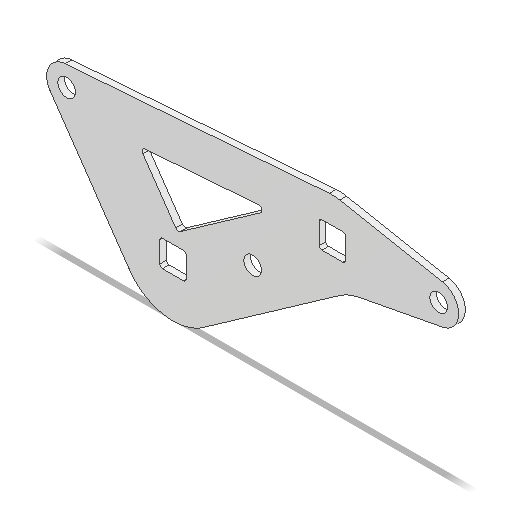
# Autodesk Inventor part: Gearbox
Saved by Autodesk Inventor 2025.2 (Build 292293000, 293)
## iProperties
Created: 2025-02-16
Part Number: Gearbox
Material: Acetal Resin, White
Document SubType Name: Modeling
Designer: avere
Density: 1.425 g/cm^3
Appearance: Smooth - White
Author: avere
Autodesk Inventor part; units mm, degrees
ref_plane "YZ Plane" through (0, 0, 0) normal (1, 0, 0) x (0, 1, 0)
ref_plane "XZ Plane" through (0, 0, 0) normal (0, 1, 0) x (-1, 0, 0)
ref_plane "XY Plane" through (0, 0, 0) normal (0, 0, 1) x (1, 0, 0)
sketch "Sketch1" plane through (0, 0, 0) normal (0, 0, 1) x (1, 0, 0)
  line L0 (35.5854, -19.7457) -> (40.6146, -19.7457)
  line L1 (41.2496, -20.3807) -> (41.2496, -25.4099)
  line L2 (40.6146, -26.0449) -> (35.5854, -26.0449)
  line L3 (34.9504, -25.4099) -> (34.9504, -20.3807)
  line L4 (34.9504, -19.7457) -> (41.2496, -26.0449) construction
  line L5 (41.2496, -19.7457) -> (34.9504, -26.0449) construction
  line L6 (73.6854, 3.1496) -> (78.7146, 3.1496)
  line L7 (79.3496, 2.5146) -> (79.3496, -2.5146)
  line L8 (78.7146, -3.1496) -> (73.6854, -3.1496)
  line L9 (73.0504, -2.5146) -> (73.0504, 2.5146)
  line L10 (73.0504, 3.1496) -> (79.3496, -3.1496) construction
  line L11 (79.3496, 3.1496) -> (73.0504, -3.1496) construction
  arc A0 (35.5854, -19.7457) -> (34.9504, -20.3807) centre (35.5854, -20.3807) ccw
  arc A1 (34.9504, -25.4099) -> (35.5854, -26.0449) centre (35.5854, -25.4099) ccw
  arc A2 (40.6146, -26.0449) -> (41.2496, -25.4099) centre (40.6146, -25.4099) ccw
  arc A3 (41.2496, -20.3807) -> (40.6146, -19.7457) centre (40.6146, -20.3807) ccw
  arc A4 (73.0504, -2.5146) -> (73.6854, -3.1496) centre (73.6854, -2.5146) ccw
  arc A5 (73.6854, 3.1496) -> (73.0504, 2.5146) centre (73.6854, 2.5146) ccw
  arc A6 (79.3496, 2.5146) -> (78.7146, 3.1496) centre (78.7146, 2.5146) ccw
  arc A7 (78.7146, -3.1496) -> (79.3496, -2.5146) centre (78.7146, -2.5146) ccw
  arc A8 (12.3428, 4.7491) -> (8.7773, -2.7007) centre (12.7, 0) ccw
  arc A9 (77.9859, 9.3561) -> (75.4856, 9.4982) centre (76.2, 0) ccw
  arc A10 (27.6395, -30.0972) -> (45.4023, -33.2859) centre (38.1, -22.8953) ccw
  line L12 (12.3428, 4.7491) -> (75.4856, 9.4982)
  line L13 (8.7773, -2.7007) -> (27.6395, -30.0972)
  line L14 (45.4023, -33.2859) -> (77.7633, -10.5433)
  circle A11 centre (12.7, 0) radius 2.0955
  circle A12 centre (101.6, 0) radius 2.0955
  arc A13 (102.493, -4.678) -> (102.493, 4.678) centre (101.6, 0) ccw
  line L15 (77.9859, 9.3561) -> (102.493, 4.678)
  line L16 (102.493, -4.678) -> (82.6844, -8.4592)
  arc A14 (82.6844, -8.4592) -> (77.7633, -10.5433) centre (85.0656, -20.934) ccw
  line L17 (31.4974, -3.3622) -> (58.4855, -1.3323)
  line L18 (39.8718, -16.2172) -> (59.0014, -2.7733)
  line L19 (30.9032, -4.6038) -> (38.7616, -16.0179)
  arc A15 (31.4974, -3.3622) -> (30.9032, -4.6038) centre (31.5569, -4.1537) ccw
  arc A16 (38.7616, -16.0179) -> (39.8718, -16.2172) centre (39.4154, -15.5677) ccw
  arc A17 (59.0014, -2.7733) -> (58.4855, -1.3323) centre (58.545, -2.1239) ccw
  circle A18 centre (57.15, -14.5521) radius 2.0955
  point P0 (76.2, 0)
  point P1 (79.9995, -8.9717)
  point P2 (38.1, -22.8953)
  dimension "d7" = 6.2992
  dimension "d8" = 6.2992
  dimension "d12" = 6.2992
  dimension "d13" = 6.2992
  dimension "d16" = 19.05
  dimension "d17" = 25.4
  dimension "d21" = 4.191
  dimension "d22" = 63.5
  dimension "d23" = 4.7625
  dimension "d24" = 4.191
  dimension "d25" = 9.525
  dimension "d26" = 25.4
  dimension "d27" = 12.7
  dimension "d28" = 9.525
  dimension "d31" = 17.145
  dimension "d32" = 17.145
  dimension "d33" = 0.7937
  dimension "d34" = 4.191
  dimension "d38" = 8.5725
  constraints: 40 end point, 34 tangent, 32 point on circle, 19 centre point, 18 point on line, 9 equal radius, 7 parallel, 4 midpoint, 3 coincident, 2 horizontal, 2 horizontal alignment, 2 perpendicular, 2 other
  measures "d7" distance of L10.end L11.end
  measures "d8" distance of L11.start L10.end
  measures "d12" distance of L5.end L4.start
  measures "d13" distance of L4.end L5.end
  measures "d16" diameter of A9
  measures "d17" diameter of A10
  measures "d21" diameter of A11
  measures "d22" distance of A9.centre A8.centre
  measures "d23" radius of A8
  measures "d24" diameter of A12
  measures "d25" diameter of A13
  measures "d26" distance of A12.centre A9.centre
  measures "d27" radius of A14
  measures "d28" distance between parallel lines of L17 L12
  measures "d31" distance between parallel lines of L14 L18
  measures "d32" distance between parallel lines of L13 L19
  measures "d33" radius of A15
  measures "d34" diameter of A18
  measures "d38" distance from line of L18 A18.centre
extrude "Extrusion1" add sketch "Sketch1" along normal blind 1.5875
body "Solid1"
